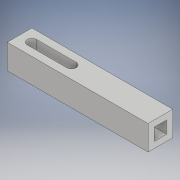
# Autodesk Inventor part: Arm_v2_richard
Saved by Autodesk Inventor 2018 (Build 220112000, 112)
## iProperties
Created: 2017-05-03
Part Number: Arm_v2_richard
Material: Generic
Document SubType Name: Modeling
Designer: mundhend06
Density: 1 g/cm^3
Appearance: Default
Author: mundhend06
Autodesk Inventor part; units mm, degrees
ref_plane "YZ Plane" through (0, 0, 0) normal (1, 0, 0) x (0, 1, 0)
ref_plane "XZ Plane" through (0, 0, 0) normal (0, 1, 0) x (-1, 0, 0)
ref_plane "XY Plane" through (0, 0, 0) normal (0, 0, 1) x (1, 0, 0)
sketch "Sketch1" plane through (0, 0, 0) normal (0, 1, 0) x (-1, 0, 0)
  line L0 (50, 80) -> (-50, 80) construction
  line L1 (-50, 80) -> (-50, -80) construction
  line L2 (-50, -80) -> (50, -80) construction
  line L3 (50, -80) -> (50, 80) construction
  line L4 (50, -80) -> (40, -80)
  line L5 (40, -80) -> (40, -50)
  line L6 (50, -80) -> (50, -50)
  line L7 (-50, 80) -> (-50, 60)
  line L8 (-50, 80) -> (-40, 80)
  line L9 (-40, 80) -> (-40, 60)
  line L10 (-40, 60) -> (50, -50)
  line L11 (-50, 60) -> (40, -50)
  point P0 (0, 0)
  point P1 (50, 0)
  point P2 (0, -80)
  dimension "d0" = 160
  dimension "d1" = 100
  dimension "d2" = 10
  dimension "d3" = 30
  dimension "d4" = 20
  dimension "d5" = 10
  constraints: 24 end point, 4 point on line, 3 perpendicular, 2 midpoint, 2 parallel, 1 horizontal, 1 horizontal alignment, 1 vertical alignment
  measures "d0" distance of L2.end L0.start
  measures "d1" distance of L1.end L2.end
  measures "d2" distance of L2.end L4.end
  measures "d3" distance of L4.end L5.end
  measures "d4" distance of L0.end L7.end
  measures "d5" distance of L0.end L8.end
extrude "Extrusion1" add sketch "Sketch1" along normal blind 10
sketch "Sketch2" plane through (40, 0, 80) normal (0, 0, 1) x (1, 0, 0)
  line L0 (-90, 0) -> (0, 0) construction
  line L1 (10, 10) -> (-80, 10) construction
  line L2 (0, 0) -> (10, 10) construction
  line L3 (2.5, 7.5) -> (7.5, 7.5)
  line L4 (7.5, 7.5) -> (7.5, 2.5)
  line L5 (7.5, 2.5) -> (2.5, 2.5)
  line L6 (2.5, 2.5) -> (2.5, 7.5)
  line L7 (2.5, 7.5) -> (7.5, 2.5) construction
  line L8 (7.5, 7.5) -> (2.5, 2.5) construction
  point P0 (-40, 0)
  point P1 (5, 5)
  dimension "d8" = 5
  dimension "d9" = 5
  constraints: 14 end point, 3 midpoint, 2 parallel, 1 horizontal, 1 perpendicular
  measures "d8" distance of L4.end L5.end
  measures "d9" distance of L3.end L4.end
extrude "Extrusion2" cut sketch "Sketch2" against normal blind 15
sketch "Sketch4" plane through (0, 10, 0) normal (0, 1, 0) x (1, 0, 0)
  line L0 (50, -80) -> (50, -60) projected
  line L1 (50, -60) -> (-84.9338, -60)
  line L2 (-84.9338, -60) -> (-84.9338, 89.9806)
  line L3 (-84.9338, 89.9806) -> (50, 89.9806)
  line L4 (50, 89.9806) -> (50, -60)
  point P0 (0, 0)
  constraints: 8 end point, 2 parallel, 1 horizontal, 1 perpendicular
extrude "Extrusion4" cut sketch "Sketch4" against normal blind 10
sketch "Sketch5" plane through (50, 10, 60) normal (0, 0, -1) x (-1, 0, 0)
  line L0 (0, -10) -> (0, 0) projected
  line L1 (10, -10) -> (10, 0) projected
  line L2 (0, -10) -> (10, -10)
  line L3 (10, -10) -> (10, 0)
  line L4 (10, 0) -> (0, 0)
  line L5 (0, 0) -> (0, -10)
  point P0 (50, -10)
  constraints: 8 end point, 2 parallel, 1 horizontal, 1 perpendicular
extrude "Extrusion5" add sketch "Sketch5" along normal blind 10
sketch "Sketch7" plane through (50, 10, 50) normal (0, 0, -1) x (-1, 0, 0)
  line L0 (0, 0) -> (0, -10) projected
  line L1 (10, 0) -> (0, 0) projected
  line L2 (0, -10) -> (10, -10)
  line L3 (10, -10) -> (10, 0)
  line L4 (10, 0) -> (0, 0)
  line L5 (0, 0) -> (0, -10)
  point P0 (50, -10)
  constraints: 8 end point, 2 parallel, 1 horizontal, 1 perpendicular
extrude "Extrusion6" add sketch "Sketch7" along normal blind 27
sketch "Sketch9" plane through (0, 10, 0) normal (0, 1, 0) x (1, 0, 0)
  arc A0 (46.9, -28) -> (43.1, -28) centre (45, -28) ccw
  line L0 (40, -23) -> (50, -23) projected
  arc A1 (43.1, -44) -> (46.9, -44) centre (45, -44) ccw
  line L1 (40, -80) -> (40, -23) projected
  line L2 (43.1, -44) -> (43.1, -28)
  line L3 (46.9, -44) -> (46.9, -28)
  point P0 (0, 0)
  dimension "d25" = 3.8
  dimension "d26" = 5
  dimension "d27" = 3.8
  dimension "d28" = 16
  dimension "d29" = 5
  constraints: 4 end point, 4 point on circle, 2 centre point, 2 tangent, 1 parallel, 1 vertical
  measures "d25" diameter of A0
  measures "d26" distance from line of L0 A0.centre
  measures "d27" diameter of A1
  measures "d28" distance of A0.centre A1.centre
  measures "d29" distance from line of L1 A1.centre
extrude "Extrusion7" cut sketch "Sketch9" against normal blind 5
body "Solid1"
